Autodesk Inventor part; units mm, degrees
(part 3 of 3)
  spline S229 degree 2 poles (-66.4601, 1.5815) (-66.0805, 1.7039) (-65.8968, 1.9978) knots 0 0 0 1 1 1
  line L1342 (-65.8968, 1.9978) -> (-65.5417, 2.0957)
  line L1343 (-65.5417, 2.0957) -> (-65.5907, 2.1447)
  line L1344 (-65.5907, 2.1447) -> (-65.4805, 2.2794)
  spline S230 degree 2 poles (-65.4805, 2.2794) (-65.3336, 2.3774) (-65.2968, 2.4631) knots 0 0 0 1 1 1
  line L1345 (-65.2968, 2.4631) -> (-65.0764, 2.5366)
  line L1346 (-65.0764, 2.5366) -> (-65.0152, 2.6835)
  spline S231 degree 2 poles (-65.0152, 2.6835) (-64.905, 2.6835) (-64.905, 2.7937) knots 0 0 0 1 1 1
  spline S232 degree 2 poles (-64.905, 2.7937) (-64.7703, 3.0264) (-64.2315, 3.1733) knots 0 0 0 1 1 1
  spline S233 degree 2 poles (-64.2315, 3.1733) (-64.1336, 3.1243) (-64.1336, 3.0386) knots 0 0 0 1 1 1
  spline S234 degree 2 poles (-64.1336, 3.0386) (-64.1336, 2.9039) (-64.4029, 2.1447) (-64.6233, 1.9855) knots 0 0 0 1 2 2 2
  line L1347 (-64.6233, 1.9855) -> (-65.0519, 1.6794)
  line L1348 (-65.0519, 1.6794) -> (-65.1744, 1.508)
  spline S235 degree 2 poles (-65.1744, 1.508) (-65.2478, 1.3978) (-65.3458, 1.3611) knots 0 0 0 1 1 1
  line L1349 (-65.3458, 1.3611) -> (-65.6274, 1.2386)
  line L1350 (-65.6274, 1.2386) -> (-65.8356, 1.1774)
  line L1351 (-65.8356, 1.1774) -> (-66.2887, 0.7611)
  line L1352 (-66.2887, 0.7611) -> (-66.558, 0.7366)
  line L1353 (-66.558, 0.7366) -> (-66.9131, 0.4549)
  line L1354 (-66.9131, 0.4549) -> (-67.0601, 0.308)
  spline S236 degree 2 poles (-67.0601, 0.308) (-67.0968, 0.2713) (-67.2193, 0.2223) knots 0 0 0 1 1 1
  line L1355 (-67.2193, 0.2223) -> (-68.1744, -0.1573)
  line L1356 (-68.1744, -0.1573) -> (-68.3948, -0.1818)
  line L1357 (-68.3948, -0.1818) -> (-68.5785, -0.3165)
  line L1358 (-68.5785, -0.3165) -> (-68.9336, -0.0838)
  line L1359 (-68.9336, -0.0838) -> (-69.0315, 0.3815)
  line L1360 (-69.0315, 0.3815) -> (-69.154, 0.6264)
  spline S237 degree 2 poles (-69.154, 0.6264) (-69.2029, 0.7366) (-69.4601, 2.2427) knots 0 0 0 1 1 1
  spline S238 degree 2 poles (-69.4601, 2.2427) (-69.4356, 2.3039) (-69.3131, 2.5121) knots 0 0 0 1 1 1
  line L1361 (-69.3131, 2.5121) -> (-69.3131, 2.7815)
  line L1362 (-69.3131, 2.7815) -> (-69.1295, 2.8549)
  line L1363 (-69.1295, 2.8549) -> (-68.8968, 3.4917)
  line L1364 (-68.8968, 3.4917) -> (-68.9825, 3.6998)
  spline S239 degree 2 poles (-68.9825, 3.6998) (-68.6642, 3.7611) (-68.6029, 3.8223) (-68.6029, 3.859) knots 0 0 0 1 2 2 2
  spline S240 degree 2 poles (-68.6029, 3.859) (-68.6029, 3.8957) (-68.6764, 4.0427) knots 0 0 0 1 1 1
  line L1365 (-68.6764, 4.0427) -> (-68.4315, 4.7896)
  line L1366 (-68.4315, 4.7896) -> (-68.358, 5.4631)
  line L1367 (-68.358, 5.4631) -> (-68.0152, 6.3815)
  spline S241 degree 2 poles (-68.0152, 6.3815) (-68.0397, 6.5529) (-68.4193, 6.8713) (-68.6029, 6.908) knots 0 0 0 1 2 2 2
  line L1368 (-68.6029, 6.908) -> (-68.8968, 6.7243)
  line L1369 (-68.8968, 6.7243) -> (-68.9948, 6.7243)
  spline S242 degree 2 poles (-68.9948, 6.7243) (-69.2152, 6.7243) (-69.3989, 6.8223) (-69.4111, 6.8223) knots 0 0 0 1 2 2 2
  spline S243 degree 2 poles (-69.4111, 6.8223) (-69.4723, 6.8223) (-69.5825, 6.7488) knots 0 0 0 1 1 1
  spline S244 degree 2 poles (-69.5825, 6.7488) (-69.656, 6.5896) (-69.7662, 6.5896) knots 0 0 0 1 1 1
  line L1370 (-69.7662, 6.5896) -> (-69.7907, 6.5896)
  spline S245 degree 2 poles (-69.7907, 6.5896) (-69.8397, 6.5774) (-69.9254, 6.5774) knots 0 0 0 1 1 1
  spline S246 degree 2 poles (-69.9254, 6.5774) (-70.0111, 6.5774) (-70.2193, 6.6141) knots 0 0 0 1 1 1
  spline S247 degree 2 poles (-70.2193, 6.6141) (-70.3785, 7.0304) (-70.3785, 7.1284) knots 0 0 0 1 1 1
  spline S248 degree 2 poles (-70.3785, 7.1284) (-70.3785, 7.2141) (-70.158, 7.7162) (-70.0356, 7.7162) knots 0 0 0 1 2 2 2
  line L1371 (-70.0356, 7.7162) -> (-69.9254, 7.7039)
  line L1372 (-69.9254, 7.7039) -> (-69.705, 7.7651)
  spline S249 degree 2 poles (-69.705, 7.7651) (-69.4968, 7.8264) (-69.4111, 7.8264) knots 0 0 0 1 1 1
  line L1373 (-69.4111, 7.8264) -> (-69.3621, 7.8264)
  spline S250 degree 2 poles (-69.3621, 7.8264) (-69.3376, 7.8019) (-69.2764, 7.8019) knots 0 0 0 1 1 1
  spline S251 degree 2 poles (-69.2764, 7.8019) (-69.2029, 7.8019) (-69.0805, 7.8631) (-69.007, 7.8631) knots 0 0 0 1 2 2 2
  spline S252 degree 2 poles (-69.007, 7.8631) (-68.9091, 7.8631) (-68.8723, 7.8386) knots 0 0 0 1 1 1
  line L1374 (-68.8723, 7.8386) -> (-68.5907, 7.9855)
  line L1375 (-68.5907, 7.9855) -> (-68.505, 7.9855)
  spline S253 degree 2 poles (-68.505, 7.9855) (-68.3948, 7.9855) (-68.2111, 8.0468) (-68.0764, 8.3284) knots 0 0 0 1 2 2 2
  line L1376 (-68.0764, 8.3284) -> (-67.905, 8.2917)
  spline S254 degree 2 poles (-67.905, 8.2917) (-67.8805, 8.4386) (-67.7213, 8.7447) knots 0 0 0 1 1 1
  spline S255 degree 2 poles (-67.7213, 8.7447) (-67.5866, 8.7447) (-67.5866, 8.9651) knots 0 0 0 1 1 1
  line L1377 (-67.5866, 8.9651) -> (-67.5866, 9.0508)
  line L1378 (-67.5866, 9.0508) -> (-67.6233, 8.9896)
  spline S256 degree 2 poles (-67.6233, 8.9896) (-67.5131, 9.2835) (-67.4397, 9.4427) knots 0 0 0 1 1 1
  line L1379 (-67.4397, 9.4427) -> (-67.4764, 9.7366)
  line L1380 (-67.4764, 9.7366) -> (-67.158, 10.3611)
  spline S257 degree 2 poles (-67.158, 10.3611) (-67.0233, 10.557) (-66.8029, 10.6059) knots 0 0 0 1 1 1
  spline S258 degree 2 poles (-66.8029, 10.6059) (-66.6438, 10.8386) (-65.9336, 11.2794) (-65.8233, 11.2794) knots 0 0 0 1 2 2 2
  spline S259 degree 2 poles (-65.8233, 11.2794) (-65.554, 11.2794) (-65.4927, 11.0345) knots 0 0 0 1 1 1
  line L1381 (-65.4927, 11.0345) -> (-65.7131, 10.6059)
  line L1382 (-65.7131, 10.6059) -> (-65.7131, 10.2141)
  line L1383 (-59.1499, 8.3039) -> (-58.758, 8.3039)
  line L1384 (-58.758, 8.3039) -> (-58.5131, 8.1937)
  spline S260 degree 2 poles (-58.5131, 8.1937) (-58.4152, 7.7896) (-58.2193, 7.7896) knots 0 0 0 1 1 1
  spline S261 degree 2 poles (-58.2193, 7.7896) (-58.1336, 7.7896) (-58.1336, 7.9488) knots 0 0 0 1 1 1
  spline S262 degree 2 poles (-58.1336, 7.9488) (-57.9009, 8.1202) (-57.705, 8.1202) knots 0 0 0 1 1 1
  spline S263 degree 2 poles (-57.705, 8.1202) (-57.5825, 8.1202) (-57.4233, 7.9488) (-57.4111, 7.8631) knots 0 0 0 1 2 2 2
  line L1385 (-57.4111, 7.8631) -> (-57.3499, 7.0059)
  line L1386 (-57.3499, 7.0059) -> (-57.3989, 6.8223)
  spline S264 degree 2 poles (-57.3989, 6.8223) (-57.4478, 6.6508) (-57.4968, 6.259) (-57.5948, 6.0264) (-57.6193, 6.0019) knots 0 0 0 1 2 3 3 3
  line L1387 (-57.6193, 6.0019) -> (-58.2315, 5.3529)
  line L1388 (-58.2315, 5.3529) -> (-58.158, 4.8998)
  line L1389 (-58.158, 4.8998) -> (-58.3172, 4.6304)
  line L1390 (-58.3172, 4.6304) -> (-58.3907, 4.3978)
  line L1391 (-58.3907, 4.3978) -> (-58.8682, 3.8468)
  line L1392 (-58.8682, 3.8468) -> (-59.1009, 3.259)
  spline S265 degree 2 poles (-59.1009, 3.259) (-59.3213, 3.0141) (-59.7131, 2.8794) knots 0 0 0 1 1 1
  line L1393 (-59.7131, 2.8794) -> (-59.8111, 2.4508)
  line L1394 (-59.8111, 2.4508) -> (-60.2519, 2.1692)
  line L1395 (-60.2519, 2.1692) -> (-60.6438, 1.7039)
  line L1396 (-60.6438, 1.7039) -> (-61.3417, 1.1774)
  line L1397 (-61.3417, 1.1774) -> (-61.5499, 1.1284)
  line L1398 (-61.5499, 1.1284) -> (-62.3336, 0.4794)
  line L1399 (-62.3336, 0.4794) -> (-62.554, 0.6876)
  spline S266 degree 2 poles (-62.554, 0.6876) (-62.8111, 0.8835) (-63.0193, 1.1651) (-63.0193, 1.2876) knots 0 0 0 1 2 2 2
  spline S267 degree 2 poles (-63.0193, 1.2876) (-63.0193, 1.3366) (-62.9703, 1.3855) knots 0 0 0 1 1 1
  line L1400 (-62.9703, 1.3855) -> (-62.8968, 2.0345)
  line L1401 (-62.8968, 2.0345) -> (-63.2274, 2.5733)
  spline S268 degree 2 poles (-63.2274, 2.5733) (-63.2642, 2.6345) (-63.2642, 2.6957) knots 0 0 0 1 1 1
  spline S269 degree 2 poles (-63.2642, 2.6957) (-63.2642, 2.7815) (-63.1784, 2.9039) knots 0 0 0 1 1 1
  line L1402 (-63.1784, 2.9039) -> (-63.1784, 2.9284)
  line L1403 (-63.1784, 2.9284) -> (-63.0438, 3.0508)
  line L1404 (-63.0438, 3.0508) -> (-63.1907, 3.4304)
  line L1405 (-63.1907, 3.4304) -> (-63.1417, 4.2141)
  line L1406 (-63.1417, 4.2141) -> (-63.1417, 4.4223)
  line L1407 (-63.1417, 4.4223) -> (-63.0315, 4.4835)
  spline S270 degree 2 poles (-63.0315, 4.4835) (-63.1172, 4.6304) (-63.1172, 4.8386) knots 0 0 0 1 1 1
  spline S271 degree 2 poles (-63.1172, 4.8386) (-63.1172, 4.9488) (-63.0193, 5.0713) knots 0 0 0 1 1 1
  line L1408 (-63.0193, 5.0713) -> (-62.8846, 5.0713)
  line L1409 (-62.8846, 5.0713) -> (-63.007, 5.1815)
  line L1410 (-63.007, 5.1815) -> (-62.9091, 5.3529)
  line L1411 (-62.9091, 5.3529) -> (-62.7499, 5.757)
  line L1412 (-62.7499, 5.757) -> (-62.5295, 6.0386)
  line L1413 (-62.5295, 6.0386) -> (-62.456, 6.2468)
  line L1414 (-62.456, 6.2468) -> (-62.2233, 6.5651)
  spline S272 degree 2 poles (-62.2233, 6.5651) (-62.1989, 6.6631) (-62.1744, 6.7488) knots 0 0 0 1 1 1
  line L1415 (-62.1744, 6.7488) -> (-62.1744, 6.7366)
  spline S273 degree 2 poles (-62.1744, 6.7366) (-62.1744, 6.859) (-62.0519, 7.0059) (-61.9295, 7.2141) knots 0 0 0 1 2 2 2
  line L1416 (-61.9295, 7.2141) -> (-61.5621, 7.41)
  line L1417 (-61.5621, 7.41) -> (-61.5254, 7.508)
  spline S274 degree 2 poles (-61.5254, 7.508) (-61.1458, 7.8141) (-60.7784, 7.8876) knots 0 0 0 1 1 1
  line L1418 (-60.7784, 7.8876) -> (-60.2764, 7.9855)
  line L1419 (-60.2764, 7.9855) -> (-59.9336, 8.1815)
  line L1420 (-59.9336, 8.1815) -> (-59.6764, 8.1692)
  line L1421 (-59.6764, 8.1692) -> (-59.1499, 8.3039)
  line L1422 (-59.6152, 6.9447) -> (-59.6519, 6.8835)
  spline S275 degree 2 poles (-59.6519, 6.8835) (-59.7866, 6.8835) (-59.9091, 6.8835) (-60.0193, 6.7855) knots 0 0 0 1 2 2 2
  line L1423 (-60.0193, 6.7855) -> (-60.2397, 6.8713)
  line L1424 (-60.2397, 6.8713) -> (-61.0723, 6.4059)
  spline S276 degree 2 poles (-61.0723, 6.4059) (-61.3907, 6.2345) (-61.8315, 5.4386) (-61.8315, 5.1815) knots 0 0 0 1 2 2 2
  spline S277 degree 2 poles (-61.8315, 5.1815) (-61.8315, 5.0223) (-61.758, 4.8998) knots 0 0 0 1 1 1
  line L1425 (-61.758, 4.8998) -> (-61.7336, 4.8998)
  spline S278 degree 2 poles (-61.7336, 4.8998) (-61.7336, 4.7284) (-61.6356, 4.2631) knots 0 0 0 1 1 1
  line L1426 (-61.6356, 4.2631) -> (-61.8315, 3.9692)
  line L1427 (-61.8315, 3.9692) -> (-61.6846, 3.7611)
  line L1428 (-61.6846, 3.7611) -> (-61.758, 3.4917)
  spline S279 degree 2 poles (-61.758, 3.4917) (-61.758, 3.4427) (-61.6356, 3.1733) (-61.6478, 3.0386) (-61.5131, 2.8427) knots 0 0 0 1 2 3 3 3
  line L1429 (-61.5131, 2.8427) -> (-61.5254, 2.6835)
  spline S280 degree 2 poles (-61.5254, 2.6835) (-61.5254, 2.2549) (-61.3295, 2.2549) knots 0 0 0 1 1 1
  spline S281 degree 2 poles (-61.3295, 2.2549) (-61.158, 2.2549) (-60.8764, 2.4998) knots 0 0 0 1 1 1
  spline S282 degree 2 poles (-60.8764, 2.4998) (-60.8152, 2.6957) (-60.607, 2.708) knots 0 0 0 1 1 1
  line L1430 (-60.607, 2.708) -> (-60.5336, 2.9406)
  spline S283 degree 2 poles (-60.5336, 2.9406) (-60.4111, 2.9529) (-60.4111, 3.0631) knots 0 0 0 1 1 1
  line L1431 (-60.4111, 3.0631) -> (-60.4111, 3.1121)
  spline S284 degree 2 poles (-60.4111, 3.1121) (-60.3744, 3.1366) (-60.2764, 3.1855) (-60.2764, 3.1978) knots 0 0 0 1 2 2 2
  spline S285 degree 2 poles (-60.2764, 3.1978) (-60.1784, 3.4917) (-59.9091, 3.859) knots 0 0 0 1 1 1
  line L1432 (-59.9091, 3.859) -> (-59.8601, 3.8345)
  line L1433 (-59.8601, 3.8345) -> (-59.8846, 3.8957)
  line L1434 (-59.8846, 3.8957) -> (-59.6519, 4.1529)
  line L1435 (-59.6519, 4.1529) -> (-59.358, 5.1325)
  line L1436 (-59.358, 5.1325) -> (-59.3091, 5.2304)
  line L1437 (-59.3091, 5.2304) -> (-59.2111, 5.2549)
  line L1438 (-59.2111, 5.2549) -> (-59.1989, 5.4264)
  line L1439 (-59.1989, 5.4264) -> (-59.1989, 5.5733)
  spline S286 degree 2 poles (-59.1989, 5.5733) (-59.1989, 5.61) (-59.0887, 5.8549) knots 0 0 0 1 1 1
  line L1440 (-59.0887, 5.8549) -> (-59.554, 6.2223)
  line L1441 (-59.554, 6.2223) -> (-59.1989, 6.3692)
  line L1442 (-59.1989, 6.3692) -> (-59.2478, 6.7855)
  line L1443 (-59.2478, 6.7855) -> (-59.1744, 6.9325)
  line L1444 (-59.1744, 6.9325) -> (-59.2723, 6.8835)
  line L1445 (-59.2723, 6.8835) -> (-59.6152, 6.9447)
  spline S287 degree 2 poles (-53.6642, 8.2917) (-53.4805, 8.2059) (-53.456, 8.0468) knots 0 0 0 1 1 1
  spline S288 degree 2 poles (-53.456, 8.0468) (-53.6642, 7.8264) (-53.6642, 7.41) knots 0 0 0 1 1 1
  line L1446 (-53.6642, 7.41) -> (-53.6642, 7.2876)
  spline S289 degree 2 poles (-53.6642, 7.2876) (-53.7376, 7.2141) (-53.7376, 7.1406) knots 0 0 0 1 1 1
  spline S290 degree 2 poles (-53.7376, 7.1406) (-53.7376, 7.0549) (-53.7009, 7.0182) knots 0 0 0 1 1 1
  line L1447 (-53.7009, 7.0182) -> (-53.6642, 7.0182)
  line L1448 (-53.6642, 7.0182) -> (-53.7009, 6.7978)
  line L1449 (-53.7009, 6.7978) -> (-53.8478, 6.7733)
  line L1450 (-53.8478, 6.7733) -> (-53.8968, 6.5162)
  line L1451 (-53.8968, 6.5162) -> (-53.9458, 6.5162)
  spline S291 degree 2 poles (-53.9458, 6.5162) (-53.9213, 6.3937) (-53.8478, 6.3447) knots 0 0 0 1 1 1
  spline S292 degree 2 poles (-53.8478, 6.3447) (-53.6519, 6.3692) (-53.2356, 6.8223) knots 0 0 0 1 1 1
  line L1452 (-53.2356, 6.8223) -> (-53.1989, 6.7978)
  line L1453 (-53.1989, 6.7978) -> (-52.4274, 7.3733)
  line L1454 (-52.4274, 7.3733) -> (-52.2805, 7.41)
  line L1455 (-52.2805, 7.41) -> (-51.9254, 7.6059)
  line L1456 (-51.9254, 7.6059) -> (-51.6438, 7.6794)
  spline S293 degree 2 poles (-51.6438, 7.6794) (-51.3866, 7.9121) (-50.8111, 7.9243) knots 0 0 0 1 1 1
  spline S294 degree 2 poles (-50.8111, 7.9243) (-50.554, 7.7774) (-50.4682, 7.7774) knots 0 0 0 1 1 1
  spline S295 degree 2 poles (-50.4682, 7.7774) (-50.3703, 7.7774) (-50.3703, 7.7162) knots 0 0 0 1 1 1
  spline S296 degree 2 poles (-50.3703, 7.7162) (-50.3703, 7.6672) (-50.4438, 7.41) knots 0 0 0 1 1 1
  line L1457 (-50.4438, 7.41) -> (-50.7744, 7.2141)
  line L1458 (-50.7744, 7.2141) -> (-50.9458, 6.9815)
  line L1459 (-50.9458, 6.9815) -> (-51.4846, 6.7366)
  line L1460 (-51.4846, 6.7366) -> (-51.6805, 6.8223)
  line L1461 (-51.6805, 6.8223) -> (-51.8274, 6.8223)
  line L1462 (-51.8274, 6.8223) -> (-51.8274, 6.7978)
  spline S297 degree 2 poles (-51.8274, 6.7978) (-52.3662, 6.5896) (-52.8193, 6.4917) knots 0 0 0 1 1 1
  spline S298 degree 2 poles (-52.8193, 6.4917) (-53.0274, 6.0753) (-54.1662, 4.7162) (-54.1784, 4.3733) knots 0 0 0 1 2 2 2
  line L1463 (-54.1784, 4.3733) -> (-54.2274, 3.2713)
  line L1464 (-54.2274, 3.2713) -> (-54.5213, 2.7815)
  line L1465 (-54.5213, 2.7815) -> (-54.4968, 2.0835)
  spline S299 degree 2 poles (-54.4968, 2.0835) (-54.5213, 1.9611) (-54.6682, 1.7039) (-54.7295, 1.4957) (-54.9131, 1.2264) knots 0 0 0 1 2 3 3 3
  line L1466 (-54.9131, 1.2264) -> (-55.0478, 1.1774)
  spline S300 degree 2 poles (-55.0478, 1.1774) (-55.0968, 1.1774) (-55.4519, 0.8957) knots 0 0 0 1 1 1
  line L1467 (-55.4519, 0.8957) -> (-55.8438, 0.8957)
  line L1468 (-55.8438, 0.8957) -> (-56.0152, 0.8345)
  line L1469 (-56.0152, 0.8345) -> (-56.2723, 1.0794)
  spline S301 degree 2 poles (-56.2723, 1.0794) (-56.2723, 1.2998) (-55.954, 1.9488) (-55.9295, 2.0957) knots 0 0 0 1 2 2 2
  spline S302 degree 2 poles (-55.9295, 2.0957) (-55.8193, 2.8549) (-55.5376, 2.9896) knots 0 0 0 1 1 1
  line L1470 (-55.5376, 2.9896) -> (-55.4519, 3.21)
  line L1471 (-55.4519, 3.21) -> (-55.4887, 3.3447)
  line L1472 (-55.4887, 3.3447) -> (-55.4274, 3.4549)
  line L1473 (-55.4274, 3.4549) -> (-55.6356, 3.7978)
  line L1474 (-55.6356, 3.7978) -> (-55.6356, 3.908)
  line L1475 (-55.6356, 3.908) -> (-55.6723, 4.5692)
  spline S303 degree 2 poles (-55.6723, 4.5692) (-55.5744, 4.6549) (-55.5376, 4.6549) knots 0 0 0 1 1 1
  spline S304 degree 2 poles (-55.5376, 4.6549) (-55.4764, 4.6549) (-55.4029, 4.5692) knots 0 0 0 1 1 1
  line L1476 (-55.4029, 4.5692) -> (-55.0968, 4.9611)
  line L1477 (-55.0968, 4.9611) -> (-55.1458, 5.2427)
  line L1478 (-55.1458, 5.2427) -> (-55.0723, 5.5733)
  line L1479 (-55.0723, 5.5733) -> (-55.256, 5.708)
  line L1480 (-55.256, 5.708) -> (-55.256, 6.4917)
  line L1481 (-55.256, 6.4917) -> (-55.5376, 6.2713)
  line L1482 (-55.5376, 6.2713) -> (-55.7091, 6.2713)
  line L1483 (-55.7091, 6.2713) -> (-55.954, 6.0998)
  line L1484 (-55.954, 6.0998) -> (-56.1989, 6.1611)
  line L1485 (-56.1989, 6.1611) -> (-56.456, 6.1243)
  spline S305 degree 2 poles (-56.456, 6.1243) (-56.6519, 6.1243) (-56.6519, 6.2713) knots 0 0 0 1 1 1
  spline S306 degree 2 poles (-56.6519, 6.2713) (-56.6519, 6.4917) (-56.1989, 7.1162) (-55.7336, 7.3733) knots 0 0 0 1 2 2 2
  line L1486 (-55.7336, 7.3733) -> (-55.7336, 7.41)
  line L1487 (-55.7336, 7.41) -> (-55.5376, 7.4345)
  spline S307 degree 2 poles (-55.5376, 7.4345) (-55.4152, 7.6549) (-55.256, 7.6549) knots 0 0 0 1 1 1
  spline S308 degree 2 poles (-55.256, 7.6549) (-55.158, 7.6917) (-54.9376, 7.9121) (-54.5458, 8.108) knots 0 0 0 1 2 2 2
  line L1488 (-54.5458, 8.108) -> (-54.3376, 7.9978)
  line L1489 (-54.3376, 7.9978) -> (-54.1784, 8.0713)
  line L1490 (-54.1784, 8.0713) -> (-53.9458, 8.1325)
  line L1491 (-53.9458, 8.1325) -> (-53.6642, 8.2917)
  constraints: 6 end point, 2 point on line, 1 horizontal, 1 parallel, 1 vertical
extrude "Extrusion3" cut sketch "Sketch3" against normal blind 1 contours L451 L452 L453 L454 L455 L3 L632 L633 L634 L635 L636 L637 L638 L0 | L0 L638 S120 L639 L640 S121 L641 L642 L643 L644 L645 L646 L647 L648 S122 L649 L650 L651 L652 L653 L654 L655 L656 S123 L657 L658 S124 L659 L660 L661 S125 L662 S126 L663 L664 L665 L666 L667 L668 L669 L670 L671 L672 L673 L674 L675 L676 L677 L678 L679 L680 L681 L682 S127 L683 L684 L685 L686 L687 L688 L689 S128 L690 L438 L439 L440 L441 L442 L443 L444 S98 L445 S99 S100 S101 L446 L447 L448 L449 L450 S102 L451 | L152 S21 L153 S22 L154 L155 L156 L157 L158 L159 L160 L161 L162 L163 L164 L165 L166 L167 L168 L169 L170 L171 S23 L172 L173 L174 L175 L176 L177 L178 L179 L180 L181 S24 L182 S25 L183 L184 L185 L186 L187 S26 L188 L189 L190 L191 L192 S27 L193 S28 L194 S0 L4 L5 S1 L6 L7 L8 L9 L10 L11 L12 L13 L14 L15 L16 L17 L18 L19 L20 L21 S2 S3 L22 L23 L24 L25 L26 S4 L27 L28 S5 L29 S6 L30 L31 L32 L33 L34 L35 L36 S7 L37 L38 L39 L40 L41 S8 L42 L43 L44 L45 L46 L47 L48 L49 L50 L51 L52 L53 L54 L55 L56 L57 L58 L59 S9 L60 L61 L62 L63 S10 L64 L65 S11 L66 L67 S12 L68 L69 L70 S13 L71 L72 L73 L74 L75 L76 L77 L78 L79 L80 L81 L82 L83 L84 L85 L86 L87 L88 S14 L89 L90 L91 L92 L93 S15 L94 L95 L96 L97 L98 L99 L100 L101 L102 L103 L104 L105 L106 S16 L107 L108 L109 L110 L111 L112 L113 L114 L115 L116 L117 L118 L119 L120 L3 L122 L123 L124 S17 L125 L126 L127 L128 S18 L129 L130 L131 L132 L133 L134 L135 L136 L137 L138 L139 L140 L141 L142 S19 L143 L144 L145 L146 L147 L148 L149 L150 L151 S20 | L3 S20 L152 | L1359 L1360 S237 S238 L1361 L1362 L1363 L1364 S239 S240 L1365 L1366 L1367 S241 L1368 L1369 S242 S243 S244 L1370 S245 S246 S247 S248 L1371 L1372 S249 L1373 S250 S251 S252 L1374 L1375 S253 L1376 S254 S255 L1377 L1378 S256 L1379 L1380 S257 S258 S259 L1381 L1382 S220 L1314 L1315 L1316 L1317 L1318 S221 L1319 S222 L1320 S223 S224 L1321 L1322 L1323 L1324 L1325 L1326 L1327 S225 L1328 S226 L1329 S227 L1330 L1331 L1332 L1333 L1334 L1335 L1336 L1337 L1338 L1339 L1340 S228 L1341 S229 L1342 L1343 L1344 S230 L1345 L1346 S231 S232 S233 S234 L1347 L1348 S235 L1349 L1350 L1351 L1352 L1353 L1354 S236 L1355 L1 | L1 L1355 L1356 L1357 L1358 L1359 | L3 L120 L121 L122 | L455 L456 L457 L458 L459 L460 L461 L462 L463 L464 L465 L466 L467 L468 L469 L470 L471 L472 L473 L474 L475 L476 L477 S103 L478 L479 L480 L481 L482 L483 L484 L485 L486 L487 L488 L489 L490 S104 L491 L492 S105 L493 S106 L494 L495 L496 L497 L498 L499 L500 L501 L502 L503 L504 L505 L506 S107 L507 L508 L509 L510 L511 L512 L513 L514 L515 L516 L517 L518 L519 S108 L520 L521 S109 L522 L523 L524 L525 L526 L527 L528 S110 L529 L530 L531 L532 L533 L534 L535 L536 L537 L538 L539 L540 L541 L542 L543 L544 S111 L545 L546 L547 L548 L549 L550 S112 L551 L552 L553 L554 L555 S113 L556 L557 L558 L559 L560 L561 S114 L562 L563 S115 L564 L565 L566 L567 L568 L569 L570 L571 L572 L573 L574 L575 L576 L577 L578 L579 L580 L581 L582 L583 S116 L584 L585 L586 L587 L588 S117 L589 L590 L591 L592 L593 L594 L595 L596 L597 L598 L599 L600 L601 L602 L603 L604 L605 L606 L607 L608 L609 L610 L611 L612 L613 L614 L615 L616 L617 L618 L619 L620 S118 L621 S119 L622 L623 L624 L625 L626 L627 L628 L629 L630 L631 L632 L3 | S68 L381 L382 L383 L384 L385 L386 L387 L388 L389 L390 L391 S69 L392 S70 S71 L393 L3 | L3 L393 L394 S72 L395 L396 L397 S73 S74 S75 L398 L399 L400 S76 S77 L401 L402 S78 L403 S79 L404 S80 S81 L405 L406 S82 S83 S84 S85 L407 S86 L408 S87 L409 L410 L411 L412 L413 L414 L415 S88 S89 L416 L417 L418 L419 S90 S91 S92 L350 L351 L352 L353 L354 L355 S57 L356 L357 L358 L359 L360 L361 L362 L363 S58 L364 L365 S59 S60 S61 L366 S62 L367 S63 S64 S65 L368 S66 L369 L370 L371 L372 S67 L373 L374 L375 L376 L377 L378 L379 L380 S68 | L269 L270 L271 S44 L272 S45 L273 L274 L275 S46 S47 L276 L277 S48 L278 L279 L280 L281 L282 S49 L283 L284 L285 L286 L287 L288 S50 L289 L290 L291 L292 L293 L294 L295 L296 L297 L298 S51 L299 L300 L301 L302 L303 S29 L195 L196 L197 L198 S30 L199 L200 S31 L201 L202 L203 L204 L205 S32 S33 S34 L206 L207 L208 S35 L209 L210 L211 L212 L213 L214 S36 L215 L216 L217 S37 L218 L219 L220 L221 L222 L223 L224 L225 L226 S38 L3 L230 L231 L232 L233 L234 S40 L235 L236 L237 L238 L239 L240 L241 L242 L243 L244 L245 S41 L246 L247 L248 S42 L249 L250 L251 L252 L253 L254 S43 L255 L256 L257 L258 L259 L260 L261 | L3 L261 L262 L263 L264 L265 L266 L267 L268 L269 | S190 L1257 L1258 L1259 L1260 L1261 L1262 L1263 L1264 L1265 L1266 L1267 S191 L1268 S192 S193 L1269 L3 | L3 L1269 L1270 S194 L1271 L1272 L1273 S195 S196 S197 L1274 L1275 L1276 S198 S199 L1277 L1278 S200 L1279 S201 L1280 S202 S203 L1281 L1282 S204 S205 S206 S207 L1283 S208 L1284 S209 L1285 L1286 L1287 L1288 L1289 L1290 L1291 S210 S211 L1292 L1293 L1294 L1295 S212 S213 S214 L1226 L1227 L1228 L1229 L1230 L1231 S179 L1232 L1233 L1234 L1235 L1236 L1237 L1238 L1239 S180 L1240 L1241 S181 S182 S183 L1242 S184 L1243 S185 S186 S187 L1244 S188 L1245 L1246 L1247 L1248 S189 L1249 L1250 L1251 L1252 L1253 L1254 L1255 L1256 S190 | L827 L828 L829 L830 L831 L832 L833 L834 L835 L836 L837 L838 L839 L840 L841 L842 L843 L844 L845 L846 L847 L848 L849 L850 L851 L852 L853 L854 L855 L856 L857 L858 L859 L860 S142 L861 L862 L863 L864 L865 L866 L867 S143 L868 L869 L870 L871 L872 S144 L873 L874 L875 L876 L877 L878 L879 L880 L691 S129 L692 L693 L694 L695 L696 L697 L698 L699 L700 S130 L701 L702 L703 L704 L705 L706 L707 L708 L709 L710 L711 L712 L713 L714 S131 L715 L716 L717 L718 L719 L720 L721 S132 L722 L723 L724 L725 L726 L727 L728 L729 L730 L731 L732 L733 S133 L734 S134 L735 L736 L737 L738 L739 L740 S135 L741 L742 L743 L744 L745 S136 L746 L747 L748 L749 L750 L751 L752 L753 L754 L755 S137 L756 L757 L758 L759 L760 L761 L762 L763 L764 L765 L766 L767 L768 L769 L770 L771 L772 L773 L774 L775 L776 L777 L778 L779 L780 L781 L782 L783 L784 L3 L788 L789 L790 L791 L792 L793 L794 L795 L796 L797 L798 L799 L800 L801 L802 L803 S138 L804 L805 L806 L807 L808 L809 L810 L811 L812 L813 L814 L815 | L3 L815 S139 S140 L816 L817 L818 L819 L820 L821 L822 L823 L824 S141 L825 L826 L827 | S38 L227 L228 L229 S39 L230 L3 | L1143 L1144 L1145 L1146 L1147 S170 L1148 L1149 L1150 L1151 L1152 L1153 L1154 L1155 L1156 S171 L1157 L1158 L1159 L1160 L1161 L1162 L1163 S172 L1164 L1165 L1166 L1167 L3 | L3 L1168 L1169 L1170 L1171 L1172 L1173 L1174 L1175 L1176 L1177 L1178 L1179 L1180 L1181 L1182 L1183 L1184 L1185 L1186 L1187 L1188 L1189 L1190 L1191 L1192 L1193 L1194 L1195 L1196 L1197 L1198 L1199 L1200 L1201 L1202 S173 L1203 S174 L1204 L1205 L1206 L1207 L1208 L1064 L1065 L1066 L1067 L1068 L1069 L1070 L1071 L1072 L1073 L1074 L1075 L1076 L1077 L1078 L1079 L1080 L1081 L1082 L1083 L1084 L1085 L1086 L1087 L1088 S163 L1089 L1090 L1091 L1092 L1093 L1094 L1095 L1096 L1097 L1098 L1099 L1100 L1101 L1102 L1103 S164 L1104 L1105 L1106 L1107 L1108 S165 L1109 L1110 S166 L1111 L1112 L1113 L1114 L1115 L1116 L1117 L1118 L1119 L1120 L1121 L1122 L1123 L1124 S167 L1125 L1126 L1127 L1128 S168 L1129 L1130 L1131 L1132 L1133 L1134 L1135 L1136 L1137 L1138 L1139 L1140 L1141 S169 L1142 L1143 | L3 L785 L786 L787 L788 | L918 L919 L920 L921 L922 L923 L3 | L3 L923 L924 L925 L926 L927 L928 L929 L930 L931 S148 L932 L933 L934 L935 S149 L936 L937 L938 L939 L940 L941 L942 L943 L944 S150 L945 L946 L947 S151 L948 L949 L950 L951 L952 L953 L954 L955 L956 L957 L958 L959 L960 L961 L962 L963 L964 L965 L976 L977 L978 L979 L980 L981 L982 L983 L984 L985 L986 L987 L988 L989 L990 L991 L992 L993 L994 S152 L995 L996 L997 L998 L999 L1000 L1001 L1002 L1003 L1004 L1005 L1006 L1007 L1008 L1009 L1010 L1011 L1012 L1013 L1014 L1015 S153 L1016 L1017 L1018 L1019 S154 L1020 L1021 L1022 S155 L1023 L1024 L1025 L1026 L1027 L1028 S156 L1029 L1030 L1031 L1032 L1033 L1034 L1035 L1036 L1037 L1038 L1039 L1040 L1041 L1042 L1043 L1044 L1045 L1046 L1047 S157 L1048 L1049 L1050 L1051 S158 S159 L1052 L1053 S160 L1054 L1055 L1056 L1057 L1058 S161 L1059 L1060 L1061 L1062 S162 L1063 L881 L882 L883 L884 L885 L886 L887 L888 L889 L890 L891 L892 L893 L894 L895 L896 L897 L898 S145 L899 L900 L901 S146 L902 L903 L904 L905 L906 L907 L908 L909 L910 S147 L911 L912 L913 L914 L915 L916 L917 L918 | L3 L965 L966 L967 L968 L969 L970 L971 L972 L973 L974 L975 | L420 L421 L422 S93 L423 S94 L424 L425 S95 S96 L426 L427 L428 L429 L430 L431 S97 L432 L433 L434 L435 L436 L437 | L1296 L1297 L1298 S215 L1299 S216 L1300 L1301 S217 S218 L1302 L1303 L1304 L1305 L1306 L1307 S219 L1308 L1309 L1310 L1311 L1312 L1313 | L1383 L1384 S260 S261 S262 S263 L1385 L1386 S264 L1387 L1388 L1389 L1390 L1391 L1392 S265 L1393 L1394 L1395 L1396 L1397 L1398 L1399 S266 S267 L1400 L1401 S268 S269 L1402 L1403 L1404 L1405 L1406 L1407 S270 S271 L1408 L1409 L1410 L1411 L1412 L1413 L1414 S272 S273 L1416 L1417 S274 L1418 L1419 L1420 L1421 | S287 S288 L1446 S289 S290 L1447 L1448 L1449 L1450 L1451 S291 S292 L1452 L1453 L1454 L1455 L1456 S293 S294 S295 S296 L1457 L1458 L1459 L1460 L1461 L1462 S297 S298 L1463 L1464 L1465 S299 L1466 S300 L1467 L1468 L1469 S301 S302 L1470 L1471 L1472 L1473 L1474 L1475 S303 S304 L1476 L1477 L1478 L1479 L1480 L1481 L1482 L1483 L1484 L1485 S305 S306 L1486 L1487 S307 S308 L1488 L1489 L1490 L1491
body "Solid1"
